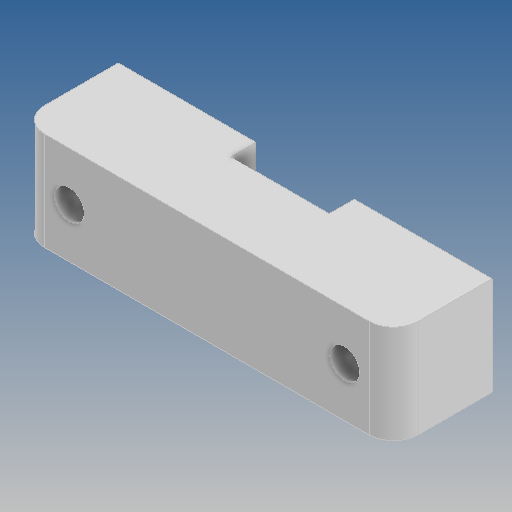
# Autodesk Inventor part: 0008-30-013
Saved by Autodesk Inventor 2020 (Build 240168000, 168)
## iProperties
Created: 2021-06-01
Part Number: 0008-30-013
Material: Generic
Document SubType Name: Modeling
Designer: Iulian Bors
Density: 1 g/cm^3
Appearance: Default
Author: Iulian Bors
Subject: 013
Autodesk Inventor part; units mm, degrees
ref_plane "YZ Plane" through (0, 0, 0) normal (1, 0, 0) x (0, 1, 0)
ref_plane "XZ Plane" through (0, 0, 0) normal (0, 1, 0) x (-1, 0, 0)
ref_plane "XY Plane" through (0, 0, 0) normal (0, 0, 1) x (1, 0, 0)
sketch "Sketch1" plane through (0, 0, 0) normal (0, 0, 1) x (1, 0, 0)
  line L0 (-38, 10) -> (38, 10)
  line L1 (38, 10) -> (38, -10)
  line L2 (38, -10) -> (-38, -10)
  line L3 (-38, -10) -> (-38, 10)
  point P0 (0, 0)
  point P1 (-38, 0)
  point P2 (0, 10)
  dimension "d0" = 76
  dimension "d1" = 20
  constraints: 8 end point, 2 midpoint, 2 parallel, 1 horizontal, 1 horizontal alignment, 1 perpendicular, 1 vertical alignment
  measures "d0" distance of L0.start L0.end
  measures "d1" distance of L2.end L0.start
extrude "Extrusion1" add sketch "Sketch1" along normal blind 20
sketch "Sketch6" plane through (0, 0, 0) normal (1, 0, 0) x (0, 1, 0)
  line L0 (12, 5.4) -> (4.47, 5.4)
  line L1 (4.47, 4.175) -> (-0.23, 4.175) projected
  line L2 (10, 0) -> (10, 20) projected
  line L3 (-10, 0) -> (-10, 20) projected
  line L4 (10, 5.1) -> (4.17, 5.1)
  line L5 (4.17, 5.1) -> (4.17, 3.875)
  line L6 (4.17, 3.875) -> (-10, 3.875)
  line L7 (10, 0) -> (-10, 0) projected
  point P0 (0, 0)
  point P1 (4.17, 0)
  dimension "d16" = 0.3
  dimension "d17" = 0.3
  dimension "d18" = 0.3
  constraints: 8 end point, 2 horizontal, 2 parallel, 2 point on line, 1 perpendicular, 2 other
  measures "d16" distance between parallel lines of L0 L4
  measures "d17" distance from line of L0.end L5
  measures "d18" distance between parallel lines of L1 L6
extrude "Extrusion5" cut sketch "Sketch6" along normal mid plane 20
sketch "Sketch7" plane through (0, 0, 20) normal (0, 0, 1) x (1, 0, 0)
  line L0 (-38, 10) -> (-38, -10) projected
  line L1 (38, -10) -> (38, 10) projected
  point P0 (0, 0)
  point P1 (28, 0)
  point P2 (-28, 0)
  dimension "d21" = 10
  dimension "d22" = 10
  constraints: 2 horizontal alignment
  measures "d21" distance from line of L0 point (-28, 0)
  measures "d22" distance from line of L1 point (28, 0)
hole "Hole1" at (-28, 0, 20) at (28, 0, 20) direction (0, 0, -1) diameter 6 end through all
fillet "Fillet3" radius 5 2 edges at (-38, 0, 20) (38, 0, 20)
equation "\"d22\" = d21"
body "Solid1"
